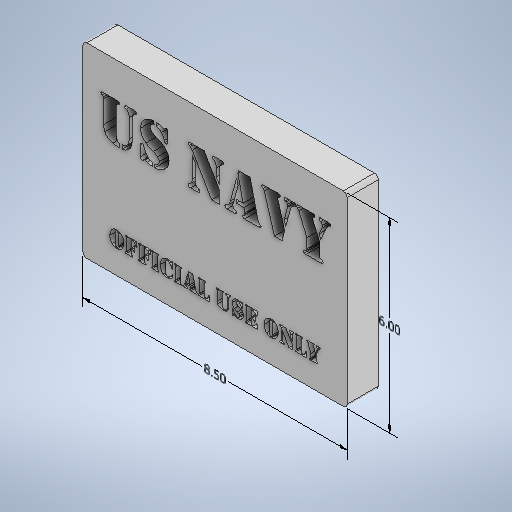
# Autodesk Inventor part: License Plate Stencil
Saved by Autodesk Inventor 2025 (Build 290162000, 162)
## iProperties
Created: 2024-06-17
Part Number: License Plate Stencil
Material: Generic
Document SubType Name: Modeling
Designer: Devon
Density: 1 g/cm^3
Appearance: Default
Author: Devon
Autodesk Inventor part; units mm, degrees
(part 1 of 2)
ref_plane "YZ Plane" through (0, 0, 0) normal (1, 0, 0) x (0, 1, 0)
ref_plane "XZ Plane" through (0, 0, 0) normal (0, 1, 0) x (-1, 0, 0)
ref_plane "XY Plane" through (0, 0, 0) normal (0, 0, 1) x (1, 0, 0)
sketch "Sketch1" plane through (0, 0, 0) normal (0, 0, 1) x (1, 0, 0)
  line L0 (0, 0) -> (304.8, 0)
  line L1 (304.8, 0) -> (304.8, 152.4)
  line L2 (304.8, 152.4) -> (0, 152.4)
  line L3 (0, 152.4) -> (0, 0)
  line L4 (0, 0) -> (44.45, 0)
  line L5 (0, 0) -> (44.45, 0) construction
  line L6 (44.45, 0) -> (44.45, 152.4)
  line L7 (304.8, 0) -> (260.35, 0)
  line L8 (260.35, 0) -> (260.35, 152.4)
  dimension "d0" = 304.8
  dimension "d1" = 152.4
  dimension "d2" = 44.45
  dimension "d3" = 0
  dimension "d4" = 44.45
  constraints: 18 end point, 3 horizontal, 3 perpendicular, 3 point on line, 2 parallel, 1 collinear
  measures "d0" distance of L2.end L1.end
  measures "d1" distance of L1.end L0.end
  measures "d2" distance of L0.start L4.end
  measures "d3" distance between parallel lines of L4 L5
  measures "d4" distance of L0.end L7.end
extrude "Extrusion1" add sketch "Sketch1" along normal blind 25.4 contours L6 L2 L8 L0
fillet "Fillet1" radius 3.175 1 edges at (260.35, 152.4, 12.7)
fillet "Fillet2" radius 3.175 1 edges at (44.45, 152.4, 12.7)
fillet "Fillet3" radius 3.175 1 edges at (260.35, 0, 12.7)
fillet "Fillet4" radius 3.175 1 edges at (44.45, 0, 12.7)
sketch "Sketch2" plane through (0, 0, 25.4) normal (0, 0, 1) x (1, 0, 0)
  line L0 (44.45, 149.225) -> (44.45, 3.175) projected
  line L1 (260.35, 3.175) -> (260.35, 149.225) projected
  line L2 (44.45, 134.9251) -> (260.35, 134.9251) construction
  line L3 (260.35, 134.9251) -> (260.35, 81.3906) construction
  line L4 (260.35, 81.3906) -> (44.45, 81.3906) construction
  line L5 (44.45, 81.3906) -> (44.45, 134.9251) construction
  line L6 (44.45, 46.9482) -> (260.35, 46.9482) construction
  line L7 (260.35, 46.9482) -> (260.35, 4.5325) construction
  line L8 (260.35, 4.5325) -> (44.45, 4.5325) construction
  line L9 (44.45, 4.5325) -> (44.45, 46.9482) construction
  line L10 (61.5459, 101.5708) -> (61.5459, 119.7885)
  spline S0 degree 2 poles (61.5459, 119.7885) (61.5459, 120.6153) (61.2703, 120.9736) knots 0 0 0 1 1 1
  spline S1 degree 2 poles (61.2703, 120.9736) (61.1325, 121.1941) (60.8845, 121.3043) (60.1128, 121.5524) knots 0 0 0 1 2 2 2
  spline S2 degree 2 poles (60.1128, 121.5524) (59.1757, 121.8556) (59.1757, 122.7926) knots 0 0 0 1 1 1
  spline S3 degree 2 poles (59.1757, 122.7926) (59.1757, 123.399) (60.0852, 124.0329) (60.912, 124.0329) knots 0 0 0 1 2 2 2
  line L11 (60.912, 124.0329) -> (61.5184, 124.0329)
  line L12 (61.5184, 124.0329) -> (71.9088, 124.0329)
  line L13 (71.9088, 124.0329) -> (72.5151, 124.0329)
  line L14 (72.5151, 124.0329) -> (73.342, 123.9502)
  spline S4 degree 2 poles (73.342, 123.9502) (73.7278, 123.8124) (74.2515, 123.206) (74.2515, 122.7926) knots 0 0 0 1 2 2 2
  spline S5 degree 2 poles (74.2515, 122.7926) (74.2515, 121.8556) (73.3144, 121.5524) knots 0 0 0 1 1 1
  spline S6 degree 2 poles (73.3144, 121.5524) (72.5427, 121.3043) (72.2946, 121.1941) (72.1568, 120.9736) knots 0 0 0 1 2 2 2
  spline S7 degree 2 poles (72.1568, 120.9736) (71.8812, 120.6153) (71.8812, 119.7885) knots 0 0 0 1 1 1
  line L15 (71.8812, 119.7885) -> (71.8812, 100.2755)
  spline S8 degree 2 poles (71.8812, 100.2755) (71.8812, 98.3187) (72.1017, 96.7477) (72.4049, 96.1138) knots 0 0 0 1 2 2 2
  spline S9 degree 2 poles (72.4049, 96.1138) (72.7081, 95.535) (73.4522, 95.0389) (74.4995, 94.7082) knots 0 0 0 1 2 2 2
  line L16 (74.4995, 94.7082) -> (74.4995, 91.649)
  line L17 (74.4995, 91.649) -> (74.0034, 91.649)
  spline S10 degree 2 poles (74.0034, 91.649) (70.9717, 91.649) (68.9598, 92.2002) knots 0 0 0 1 1 1
  spline S11 degree 2 poles (68.9598, 92.2002) (66.6171, 92.8065) (63.0893, 95.287) (62.3452, 96.8028) knots 0 0 0 1 2 2 2
  spline S12 degree 2 poles (62.3452, 96.8028) (61.5459, 98.4565) (61.5459, 101.5708) knots 0 0 0 1 1 1
  line L18 (76.6492, 91.649) -> (76.6492, 94.7082)
  spline S13 degree 2 poles (76.6492, 94.7082) (78.9643, 95.0114) (80.5353, 96.6099) knots 0 0 0 1 1 1
  spline S14 degree 2 poles (80.5353, 96.6099) (82.2992, 98.4565) (82.2992, 101.874) knots 0 0 0 1 1 1
  line L19 (82.2992, 101.874) -> (82.2992, 117.0324)
  spline S15 degree 2 poles (82.2992, 117.0324) (82.2992, 120.2295) (79.8463, 121.4973) knots 0 0 0 1 1 1
  spline S16 degree 2 poles (79.8463, 121.4973) (79.1297, 121.8556) (78.6887, 122.4068) (78.6887, 122.9029) knots 0 0 0 1 2 2 2
  spline S17 degree 2 poles (78.6887, 122.9029) (78.6887, 123.5092) (79.5707, 124.0329) (80.5904, 124.0329) knots 0 0 0 1 2 2 2
  line L20 (80.5904, 124.0329) -> (86.2679, 124.0329)
  spline S18 degree 2 poles (86.2679, 124.0329) (86.9845, 124.0329) (87.4806, 123.9502) (87.7011, 123.8124) knots 0 0 0 1 2 2 2
  spline S19 degree 2 poles (87.7011, 123.8124) (88.3074, 123.4816) (88.3074, 122.8753) knots 0 0 0 1 1 1
  spline S20 degree 2 poles (88.3074, 122.8753) (88.3074, 122.3517) (87.9492, 121.9934) knots 0 0 0 1 1 1
  spline S21 degree 2 poles (87.9492, 121.9934) (87.8114, 121.8831) (86.9294, 121.387) knots 0 0 0 1 1 1
  spline S22 degree 2 poles (86.9294, 121.387) (85.9097, 120.8083) (84.7521, 118.5207) (84.7521, 117.0324) knots 0 0 0 1 2 2 2
  line L21 (84.7521, 117.0324) -> (84.7521, 101.874)
  spline S23 degree 2 poles (84.7521, 101.874) (84.7521, 97.9604) (83.0433, 95.4523) knots 0 0 0 1 1 1
  spline S24 degree 2 poles (83.0433, 95.4523) (81.7755, 93.5782) (79.4329, 92.4758) knots 0 0 0 1 1 1
  spline S25 degree 2 poles (79.4329, 92.4758) (78.2753, 91.897) (76.6492, 91.649) knots 0 0 0 1 1 1
  line L22 (102.5288, 124.6668) -> (102.5288, 121.9934)
  spline S26 degree 2 poles (102.5288, 121.9934) (101.0956, 121.58) (99.5798, 119.9263) (99.5798, 118.7412) knots 0 0 0 1 2 2 2
  spline S27 degree 2 poles (99.5798, 118.7412) (99.5798, 117.5561) (100.8476, 115.8198) (102.2532, 115.0205) knots 0 0 0 1 2 2 2
  spline S28 degree 2 poles (102.2532, 115.0205) (103.2178, 114.4968) (106.6629, 112.981) knots 0 0 0 1 1 1
  spline S29 degree 2 poles (106.6629, 112.981) (108.7575, 112.0715) (111.0451, 110.6108) (112.0924, 109.5083) knots 0 0 0 1 2 2 2
  spline S30 degree 2 poles (112.0924, 109.5083) (114.8209, 106.642) (114.8209, 102.6457) knots 0 0 0 1 1 1
  spline S31 degree 2 poles (114.8209, 102.6457) (114.8209, 99.6691) (111.8443, 94.6806) (109.2536, 93.2475) knots 0 0 0 1 2 2 2
  spline S32 degree 2 poles (109.2536, 93.2475) (107.848, 92.5033) (104.5132, 91.649) (103.08, 91.649) knots 0 0 0 1 2 2 2
  line L23 (103.08, 91.649) -> (103.08, 94.2948)
  spline S33 degree 2 poles (103.08, 94.2948) (105.092, 94.7909) (106.8834, 96.5272) (106.8834, 98.0155) knots 0 0 0 1 2 2 2
  spline S34 degree 2 poles (106.8834, 98.0155) (106.8834, 99.5865) (105.4778, 100.7716) knots 0 0 0 1 1 1
  spline S35 degree 2 poles (105.4778, 100.7716) (104.5683, 101.5433) (101.95, 102.6733) knots 0 0 0 1 1 1
  spline S36 degree 2 poles (101.95, 102.6733) (99.1113, 103.9411) (96.9891, 105.0159) (95.9969, 105.7325) knots 0 0 0 1 2 2 2
  spline S37 degree 2 poles (95.9969, 105.7325) (91.6423, 108.8469) (91.6423, 114.0283) knots 0 0 0 1 1 1
  spline S38 degree 2 poles (91.6423, 114.0283) (91.6423, 116.6741) (93.8196, 121.1665) (95.7764, 122.5446) knots 0 0 0 1 2 2 2
  spline S39 degree 2 poles (95.7764, 122.5446) (98.5049, 124.4463) (102.5288, 124.6668) knots 0 0 0 1 1 1
  line L24 (101.3161, 94.2948) -> (101.3161, 91.649)
  spline S40 degree 2 poles (101.3161, 91.649) (99.4144, 91.649) (97.0993, 92.7238) knots 0 0 0 1 1 1
  spline S41 degree 2 poles (97.0993, 92.7238) (96.2449, 93.1372) (95.5835, 93.3577) (95.2803, 93.3577) knots 0 0 0 1 2 2 2
  spline S42 degree 2 poles (95.2803, 93.3577) (94.8393, 93.3577) (94.3708, 93.0546) (93.8472, 92.4482) knots 0 0 0 1 2 2 2
  spline S43 degree 2 poles (93.8472, 92.4482) (93.4337, 91.9521) (92.9377, 91.9521) knots 0 0 0 1 1 1
  spline S44 degree 2 poles (92.9377, 91.9521) (91.6423, 91.9521) (91.6423, 93.9641) knots 0 0 0 1 1 1
  line L25 (91.6423, 93.9641) -> (91.6423, 102.4252)
  spline S45 degree 2 poles (91.6423, 102.4252) (91.6423, 103.0591) (92.3864, 103.9686) (92.9377, 103.9962) knots 0 0 0 1 2 2 2
  spline S46 degree 2 poles (92.9377, 103.9962) (93.4613, 104.0237) (94.0401, 103.3898) (94.2606, 102.5906) knots 0 0 0 1 2 2 2
  spline S47 degree 2 poles (94.2606, 102.5906) (94.7842, 100.6062) (96.7962, 97.106) (98.1466, 95.9209) knots 0 0 0 1 2 2 2
  spline S48 degree 2 poles (98.1466, 95.9209) (99.5247, 94.6531) (101.3161, 94.2948) knots 0 0 0 1 1 1
  line L26 (104.3754, 121.9934) -> (104.3754, 124.5565)
  spline S49 degree 2 poles (104.3754, 124.5565) (105.781, 124.4463) (107.8205, 123.8951) (109.6946, 123.0958) knots 0 0 0 1 2 2 2
  spline S50 degree 2 poles (109.6946, 123.0958) (110.1631, 122.9029) (110.4663, 122.9029) knots 0 0 0 1 1 1
  spline S51 degree 2 poles (110.4663, 122.9029) (110.9073, 122.9029) (111.1278, 123.206) knots 0 0 0 1 1 1
  line L27 (111.1278, 123.206) -> (111.6239, 123.8951)
  spline S52 degree 2 poles (111.6239, 123.8951) (112.0097, 124.4187) (112.5334, 124.4187) knots 0 0 0 1 1 1
  spline S53 degree 2 poles (112.5334, 124.4187) (113.1673, 124.4187) (113.746, 123.5092) (113.746, 122.5446) knots 0 0 0 1 2 2 2
  line L28 (113.746, 122.5446) -> (113.746, 114.8551)
  spline S54 degree 2 poles (113.746, 114.8551) (113.746, 114.1661) (112.9743, 113.3117) (112.368, 113.3117) knots 0 0 0 1 2 2 2
  spline S55 degree 2 poles (112.368, 113.3117) (111.8995, 113.3117) (111.5136, 113.6149) knots 0 0 0 1 1 1
  spline S56 degree 2 poles (111.5136, 113.6149) (111.2931, 113.8078) (111.0451, 114.3315) (110.9348, 114.9654) knots 0 0 0 1 2 2 2
  spline S57 degree 2 poles (110.9348, 114.9654) (110.6868, 116.1229) (109.419, 118.5207) (108.5922, 119.4853) knots 0 0 0 1 2 2 2
  spline S58 degree 2 poles (108.5922, 119.4853) (106.911, 121.387) (104.3754, 121.9934) knots 0 0 0 1 1 1
  line L29 (143.5668, 124.0329) -> (155.9416, 102.5355)
  line L30 (155.9416, 102.5355) -> (155.9416, 92.2829)
  line L31 (155.9416, 92.2829) -> (149.6026, 92.2829)
  line L32 (149.6026, 92.2829) -> (133.8103, 119.4853)
  spline S59 degree 2 poles (133.8103, 119.4853) (133.2866, 120.3948) (132.6252, 121.0839) (132.1291, 121.2492) knots 0 0 0 1 2 2 2
  line L33 (132.1291, 121.2492) -> (131.2471, 121.58)
  spline S60 degree 2 poles (131.2471, 121.58) (130.8888, 121.6902) (130.4754, 122.2965) (130.4754, 122.6548) knots 0 0 0 1 2 2 2
  spline S61 degree 2 poles (130.4754, 122.6548) (130.4754, 123.0682) (130.8888, 123.7297) (131.2471, 123.8675) knots 0 0 0 1 2 2 2
  spline S62 degree 2 poles (131.2471, 123.8675) (131.633, 124.0329) (133.3969, 124.0329) knots 0 0 0 1 1 1
  line L34 (133.3969, 124.0329) -> (143.5668, 124.0329)
  line L35 (133.8103, 115.8473) -> (136.2632, 111.7683)
  line L36 (136.2632, 111.7683) -> (136.2632, 99.3109)
  spline S63 degree 2 poles (136.2632, 99.3109) (136.2632, 97.6848) (137.3656, 95.5902) (138.5507, 94.9011) knots 0 0 0 1 2 2 2
  line L37 (138.5507, 94.9011) -> (139.2397, 94.5153)
  spline S64 degree 2 poles (139.2397, 94.5153) (139.8461, 94.157) (139.8461, 93.468) knots 0 0 0 1 1 1
  spline S65 degree 2 poles (139.8461, 93.468) (139.8461, 92.9443) (139.4051, 92.586) knots 0 0 0 1 1 1
  spline S66 degree 2 poles (139.4051, 92.586) (139.0193, 92.2829) (137.8617, 92.2829) knots 0 0 0 1 1 1
  line L38 (137.8617, 92.2829) -> (132.5149, 92.2829)
  spline S67 degree 2 poles (132.5149, 92.2829) (130.3927, 92.2829) (130.3927, 93.4955) knots 0 0 0 1 1 1
  spline S68 degree 2 poles (130.3927, 93.4955) (130.3927, 93.9089) (130.8337, 94.405) (131.5778, 94.8185) knots 0 0 0 1 2 2 2
  spline S69 degree 2 poles (131.5778, 94.8185) (133.8103, 96.0587) (133.8103, 99.3109) knots 0 0 0 1 1 1
  line L39 (133.8103, 99.3109) -> (133.8103, 115.8473)
  line L40 (155.9416, 106.2562) -> (153.4887, 110.4178)
  line L41 (153.4887, 110.4178) -> (153.4887, 116.8671)
  spline S70 degree 2 poles (153.4887, 116.8671) (153.4887, 118.8239) (152.3587, 120.8909) (150.8979, 121.6351) knots 0 0 0 1 2 2 2
  spline S71 degree 2 poles (150.8979, 121.6351) (150.4294, 121.8556) (150.0436, 122.4068) (150.0436, 122.8202) knots 0 0 0 1 2 2 2
  spline S72 degree 2 poles (150.0436, 122.8202) (150.0436, 123.4541) (150.8704, 124.0329) (151.7799, 124.0329) knots 0 0 0 1 2 2 2
  line L42 (151.7799, 124.0329) -> (157.5676, 124.0329)
  spline S73 degree 2 poles (157.5676, 124.0329) (158.7528, 124.0329) (159.1386, 123.647) knots 0 0 0 1 1 1
  spline S74 degree 2 poles (159.1386, 123.647) (159.5245, 123.2887) (159.5245, 122.7651) knots 0 0 0 1 1 1
  spline S75 degree 2 poles (159.5245, 122.7651) (159.5245, 122.2965) (159.0835, 121.8004) (158.2567, 121.387) knots 0 0 0 1 2 2 2
  spline S76 degree 2 poles (158.2567, 121.387) (157.0164, 120.7531) (156.3825, 119.4578) knots 0 0 0 1 1 1
  spline S77 degree 2 poles (156.3825, 119.4578) (155.9416, 118.4931) (155.9416, 116.8671) knots 0 0 0 1 1 1
  line L43 (155.9416, 116.8671) -> (155.9416, 106.2562)
  line L44 (171.7063, 124.0329) -> (181.077, 124.0329)
  line L45 (181.077, 124.0329) -> (187.5262, 96.6926)
  spline S78 degree 2 poles (187.5262, 96.6926) (187.7191, 95.976) (187.9396, 95.4248) knots 0 0 0 1 1 1
  spline S79 degree 2 poles (187.9396, 95.4248) (188.1601, 94.9838) (188.8767, 94.7082) knots 0 0 0 1 1 1
  spline S80 degree 2 poles (188.8767, 94.7082) (189.483, 94.4326) (189.9515, 93.9365) (189.9515, 93.4955) knots 0 0 0 1 2 2 2
  spline S81 degree 2 poles (189.9515, 93.4955) (189.9515, 92.2829) (188.1325, 92.2829) knots 0 0 0 1 1 1
  line L46 (188.1325, 92.2829) -> (176.5294, 92.2829)
  spline S82 degree 2 poles (176.5294, 92.2829) (175.8404, 92.2829) (174.986, 92.9719) (174.986, 93.5231) knots 0 0 0 1 2 2 2
  spline S83 degree 2 poles (174.986, 93.5231) (174.986, 93.9916) (175.3719, 94.4602) (176.0058, 94.7909) knots 0 0 0 1 2 2 2
  spline S84 degree 2 poles (176.0058, 94.7909) (176.4743, 95.0389) (176.8602, 95.5902) (176.8602, 96.0036) knots 0 0 0 1 2 2 2
  spline S85 degree 2 poles (176.8602, 96.0036) (176.8602, 96.417) (176.7775, 96.7201) knots 0 0 0 1 1 1
  line L47 (176.7775, 96.7201) -> (176.0334, 100.0826)
  line L48 (176.0334, 100.0826) -> (169.5566, 100.0826)
  line L49 (169.5566, 100.0826) -> (170.1905, 102.8386)
  line L50 (170.1905, 102.8386) -> (175.3995, 102.8386)
  line L51 (175.3995, 102.8386) -> (171.1, 121.7453)
  line L52 (171.1, 121.7453) -> (171.7063, 124.0329)
  line L53 (170.0802, 118.1073) -> (171.2653, 113.3117)
  line L54 (171.2653, 113.3117) -> (167.1588, 98.2911)
  spline S86 degree 2 poles (167.1588, 98.2911) (166.9659, 97.6296) (166.9659, 97.0784) knots 0 0 0 1 1 1
  spline S87 degree 2 poles (166.9659, 97.0784) (166.9659, 95.6177) (168.3439, 94.9838) knots 0 0 0 1 1 1
  line L55 (168.3439, 94.9838) -> (169.1432, 94.598)
  spline S88 degree 2 poles (169.1432, 94.598) (169.9149, 94.2672) (169.9149, 93.4404) knots 0 0 0 1 1 1
  spline S89 degree 2 poles (169.9149, 93.4404) (169.9149, 92.2829) (168.2337, 92.2829) knots 0 0 0 1 1 1
  line L56 (168.2337, 92.2829) -> (162.3357, 92.2829)
  spline S90 degree 2 poles (162.3357, 92.2829) (161.4537, 92.2829) (160.4615, 92.9994) (160.4615, 93.6333) knots 0 0 0 1 2 2 2
  spline S91 degree 2 poles (160.4615, 93.6333) (160.4615, 94.2948) (161.4813, 94.7358) knots 0 0 0 1 1 1
  spline S92 degree 2 poles (161.4813, 94.7358) (162.4459, 95.1767) (163.3554, 95.8382) (163.7688, 96.417) knots 0 0 0 1 2 2 2
  spline S93 degree 2 poles (163.7688, 96.417) (164.4027, 97.3816) (164.8437, 98.9526) knots 0 0 0 1 1 1
  line L57 (164.8437, 98.9526) -> (170.0802, 118.1073)
  line L58 (209.2441, 100.4133) -> (207.0392, 92.2829)
  line L59 (207.0392, 92.2829) -> (200.9207, 92.2829)
  line L60 (200.9207, 92.2829) -> (192.6525, 120.0917)
  spline S94 degree 2 poles (192.6525, 120.0917) (192.4596, 120.698) (192.1564, 121.139) (191.7981, 121.3043) knots 0 0 0 1 2 2 2
  spline S95 degree 2 poles (191.7981, 121.3043) (191.054, 121.6075) (190.5854, 122.1312) (190.5854, 122.6273) knots 0 0 0 1 2 2 2
  spline S96 degree 2 poles (190.5854, 122.6273) (190.5854, 123.3438) (191.2193, 123.7297) knots 0 0 0 1 1 1
  spline S97 degree 2 poles (191.2193, 123.7297) (191.6879, 124.0329) (192.8179, 124.0329) knots 0 0 0 1 1 1
  line L61 (192.8179, 124.0329) -> (203.1531, 124.0329)
  spline S98 degree 2 poles (203.1531, 124.0329) (204.1453, 124.0329) (204.8619, 123.9502) (205.11, 123.8124) knots 0 0 0 1 2 2 2
  spline S99 degree 2 poles (205.11, 123.8124) (205.3304, 123.647) (205.6612, 123.0407) (205.6612, 122.7651) knots 0 0 0 1 2 2 2
  spline S100 degree 2 poles (205.6612, 122.7651) (205.6612, 121.8831) (204.8344, 121.5248) knots 0 0 0 1 1 1
  spline S101 degree 2 poles (204.8344, 121.5248) (204.228, 121.2217) (203.787, 120.5878) (203.787, 120.009) knots 0 0 0 1 2 2 2
  spline S102 degree 2 poles (203.787, 120.009) (203.787, 119.6231) (203.8697, 119.3475) knots 0 0 0 1 1 1
  line L62 (203.8697, 119.3475) -> (209.2441, 100.4133)
  line L63 (210.126, 103.7481) -> (208.9133, 108.1027)
  line L64 (208.9133, 108.1027) -> (211.5867, 117.9144)
  spline S103 degree 2 poles (211.5867, 117.9144) (211.8348, 118.8514) (211.8623, 119.0444) knots 0 0 0 1 1 1
  spline S104 degree 2 poles (211.8623, 119.0444) (211.9175, 119.568) (211.6419, 120.2019) knots 0 0 0 1 1 1
  spline S105 degree 2 poles (211.6419, 120.2019) (211.256, 121.0012) (210.4567, 121.2768) knots 0 0 0 1 1 1
  line L65 (210.4567, 121.2768) -> (209.685, 121.5524)
  spline S106 degree 2 poles (209.685, 121.5524) (208.7755, 121.8556) (208.7755, 122.7375) knots 0 0 0 1 1 1
  spline S107 degree 2 poles (208.7755, 122.7375) (208.7755, 123.3714) (209.7953, 124.0329) (210.7048, 124.0329) knots 0 0 0 1 2 2 2
  line L66 (210.7048, 124.0329) -> (216.4099, 124.0329)
  spline S108 degree 2 poles (216.4099, 124.0329) (217.4847, 124.0329) (217.8155, 123.8124) knots 0 0 0 1 1 1
  spline S109 degree 2 poles (217.8155, 123.8124) (218.3667, 123.4816) (218.3667, 122.8202) knots 0 0 0 1 1 1
  spline S110 degree 2 poles (218.3667, 122.8202) (218.3667, 122.3792) (218.0084, 121.8556) (217.5399, 121.6626) knots 0 0 0 1 2 2 2
  line L67 (217.5399, 121.6626) -> (216.3548, 121.1114)
  spline S111 degree 2 poles (216.3548, 121.1114) (215.6106, 120.7531) (214.2601, 118.6861) (213.8743, 117.3632) knots 0 0 0 1 2 2 2
  line L68 (213.8743, 117.3632) -> (210.126, 103.7481)
  line L69 (237.797, 106.8349) -> (237.797, 96.6926)
  spline S112 degree 2 poles (237.797, 96.6926) (237.797, 95.7831) (238.1553, 95.3972) knots 0 0 0 1 1 1
  spline S113 degree 2 poles (238.1553, 95.3972) (238.3207, 95.1767) (238.6514, 95.0389) (239.5609, 94.8185) knots 0 0 0 1 2 2 2
  spline S114 degree 2 poles (239.5609, 94.8185) (240.6909, 94.5704) (240.6909, 93.5507) knots 0 0 0 1 1 1
  spline S115 degree 2 poles (240.6909, 93.5507) (240.6909, 92.8616) (240.057, 92.5033) knots 0 0 0 1 1 1
  spline S116 degree 2 poles (240.057, 92.5033) (239.6987, 92.2829) (238.6238, 92.2829) knots 0 0 0 1 1 1
  line L70 (238.6238, 92.2829) -> (237.8246, 92.2829)
  line L71 (237.8246, 92.2829) -> (227.4342, 92.2829)
  line L72 (227.4342, 92.2829) -> (226.6625, 92.2829)
  spline S117 degree 2 poles (226.6625, 92.2829) (225.6152, 92.2829) (225.2018, 92.5585) knots 0 0 0 1 1 1
  spline S118 degree 2 poles (225.2018, 92.5585) (224.5954, 92.9443) (224.5954, 93.5507) knots 0 0 0 1 1 1
  spline S119 degree 2 poles (224.5954, 93.5507) (224.5954, 94.5704) (225.7254, 94.8185) knots 0 0 0 1 1 1
  spline S120 degree 2 poles (225.7254, 94.8185) (226.6349, 95.0389) (226.9381, 95.1767) (227.1035, 95.3972) knots 0 0 0 1 2 2 2
  spline S121 degree 2 poles (227.1035, 95.3972) (227.4617, 95.7831) (227.4617, 96.6926) knots 0 0 0 1 1 1
  line L73 (227.4617, 96.6926) -> (227.4617, 104.5474)
  line L74 (227.4617, 104.5474) -> (220.8747, 120.257)
  spline S122 degree 2 poles (220.8747, 120.257) (220.5164, 121.139) (219.8274, 121.5524) knots 0 0 0 1 1 1
  spline S123 degree 2 poles (219.8274, 121.5524) (219.2211, 121.9382) (218.8628, 122.4068) (218.8628, 122.8202) knots 0 0 0 1 2 2 2
  spline S124 degree 2 poles (218.8628, 122.8202) (218.8628, 124.0329) (220.6267, 124.0329) knots 0 0 0 1 1 1
  line L75 (220.6267, 124.0329) -> (232.0368, 124.0329)
  spline S125 degree 2 poles (232.0368, 124.0329) (232.9188, 124.0329) (233.2771, 123.8124) knots 0 0 0 1 1 1
  spline S126 degree 2 poles (233.2771, 123.8124) (233.8558, 123.4541) (233.8558, 122.8477) knots 0 0 0 1 1 1
  spline S127 degree 2 poles (233.8558, 122.8477) (233.8558, 122.1036) (233.1944, 121.6902) knots 0 0 0 1 1 1
  line L76 (233.1944, 121.6902) -> (232.5054, 121.2768)
  spline S128 degree 2 poles (232.5054, 121.2768) (232.1195, 121.0012) (232.1195, 120.5051) knots 0 0 0 1 1 1
  spline S129 degree 2 poles (232.1195, 120.5051) (232.1195, 119.9263) (232.3676, 119.3475) knots 0 0 0 1 1 1
  line L77 (232.3676, 119.3475) -> (237.797, 106.8349)
  line L78 (238.7065, 109.0398) -> (237.3836, 112.0991)
  line L79 (237.3836, 112.0991) -> (239.8365, 117.5561)
  spline S130 degree 2 poles (239.8365, 117.5561) (240.1397, 118.2727) (240.1397, 119.4578) knots 0 0 0 1 1 1
  spline S131 degree 2 poles (240.1397, 119.4578) (240.1397, 120.8083) (238.6514, 121.4146) knots 0 0 0 1 1 1
  spline S132 degree 2 poles (238.6514, 121.4146) (237.8521, 121.7178) (237.3561, 122.2139) (237.3561, 122.7375) knots 0 0 0 1 2 2 2
  spline S133 degree 2 poles (237.3561, 122.7375) (237.3561, 123.3714) (237.7695, 123.6746) knots 0 0 0 1 1 1
  spline S134 degree 2 poles (237.7695, 123.6746) (238.0451, 123.8951) (238.7341, 124.0329) (239.616, 124.0329) knots 0 0 0 1 2 2 2
  line L80 (239.616, 124.0329) -> (245.3487, 124.0329)
  spline S135 degree 2 poles (245.3487, 124.0329) (246.9748, 124.0329) (246.9748, 122.7375) knots 0 0 0 1 1 1
  spline S136 degree 2 poles (246.9748, 122.7375) (246.9748, 122.269) (246.5338, 121.7453) (245.8999, 121.4697) knots 0 0 0 1 2 2 2
  spline S137 degree 2 poles (245.8999, 121.4697) (244.7699, 120.9736) (244.2738, 120.45) knots 0 0 0 1 1 1
  spline S138 degree 2 poles (244.2738, 120.45) (243.5848, 119.7058) (243.1163, 118.7412) knots 0 0 0 1 1 1
  line L81 (243.1163, 118.7412) -> (242.5926, 117.5561)
  line L82 (242.5926, 117.5561) -> (238.7065, 109.0398)
  line L83 (72.551, 31.3407) -> (72.551, 32.3439)
  spline S139 degree 2 poles (72.551, 32.3439) (73.5542, 32.2998) (75.2188, 31.5722) (75.9354, 30.8667) knots 0 0 0 1 2 2 2
  spline S140 degree 2 poles (75.9354, 30.8667) (77.8316, 29.0146) (77.8316, 25.7293) knots 0 0 0 1 1 1
  spline S141 degree 2 poles (77.8316, 25.7293) (77.8316, 22.4992) (76.0236, 20.6912) knots 0 0 0 1 1 1
  spline S142 degree 2 poles (76.0236, 20.6912) (74.6235, 19.3022) (72.551, 19.1368) knots 0 0 0 1 1 1
  line L84 (72.551, 19.1368) -> (72.551, 20.162)
  spline S143 degree 2 poles (72.551, 20.162) (72.7935, 20.2172) (73.0581, 20.3936) (73.1683, 20.5589) knots 0 0 0 1 2 2 2
  spline S144 degree 2 poles (73.1683, 20.5589) (73.4219, 20.9448) (73.4219, 21.7165) knots 0 0 0 1 1 1
  line L85 (73.4219, 21.7165) -> (73.4219, 30.0288)
  spline S145 degree 2 poles (73.4219, 30.0288) (73.4219, 30.5249) (73.2565, 30.8115) knots 0 0 0 1 1 1
  spline S146 degree 2 poles (73.2565, 30.8115) (73.1463, 31.01) (72.8376, 31.2305) (72.551, 31.3407) knots 0 0 0 1 2 2 2
  spline S147 degree 2 poles (71.7903, 31.3407) (71.3162, 31.1643) (70.9304, 30.591) (70.9304, 30.0288) knots 0 0 0 1 2 2 2
  line L86 (70.9304, 30.0288) -> (70.9304, 21.7165)
  spline S148 degree 2 poles (70.9304, 21.7165) (70.9304, 20.9007) (71.1509, 20.5589) knots 0 0 0 1 1 1
  spline S149 degree 2 poles (71.1509, 20.5589) (71.3273, 20.2833) (71.7903, 20.162) knots 0 0 0 1 1 1
  line L87 (71.7903, 20.162) -> (71.7903, 19.1368)
  spline S150 degree 2 poles (71.7903, 19.1368) (69.7287, 19.3022) (68.3286, 20.6912) knots 0 0 0 1 1 1
  spline S151 degree 2 poles (68.3286, 20.6912) (66.5207, 22.4992) (66.5207, 25.7293) knots 0 0 0 1 1 1
  spline S152 degree 2 poles (66.5207, 25.7293) (66.5207, 27.3499) (67.4798, 29.9627) (68.4168, 30.8667) knots 0 0 0 1 2 2 2
  spline S153 degree 2 poles (68.4168, 30.8667) (69.1334, 31.5722) (70.7871, 32.2998) (71.7903, 32.3439) knots 0 0 0 1 2 2 2
  line L88 (71.7903, 32.3439) -> (71.7903, 31.3407)
  line L89 (84.0603, 32.0903) -> (84.0603, 21.1542)
  spline S154 degree 2 poles (84.0603, 21.1542) (84.0603, 20.7904) (84.2036, 20.6361) knots 0 0 0 1 1 1
  spline S155 degree 2 poles (84.2036, 20.6361) (84.2698, 20.5479) (84.4021, 20.4928) (84.7659, 20.4046) knots 0 0 0 1 2 2 2
  spline S156 degree 2 poles (84.7659, 20.4046) (85.2179, 20.3054) (85.2179, 19.8975) knots 0 0 0 1 1 1
  spline S157 degree 2 poles (85.2179, 19.8975) (85.2179, 19.6549) (84.9753, 19.5006) knots 0 0 0 1 1 1
  spline S158 degree 2 poles (84.9753, 19.5006) (84.799, 19.3903) (84.3911, 19.3903) knots 0 0 0 1 1 1
  line L90 (84.3911, 19.3903) -> (84.0714, 19.3903)
  line L91 (84.0714, 19.3903) -> (79.9152, 19.3903)
  line L92 (79.9152, 19.3903) -> (79.6727, 19.3903)
  spline S159 degree 2 poles (79.6727, 19.3903) (79.3419, 19.3903) (78.9781, 19.6439) (78.9781, 19.8754) knots 0 0 0 1 2 2 2
  spline S160 degree 2 poles (78.9781, 19.8754) (78.9781, 20.2502) (79.353, 20.3715) knots 0 0 0 1 1 1
  spline S161 degree 2 poles (79.353, 20.3715) (79.6616, 20.4818) (79.7608, 20.5259) (79.816, 20.614) knots 0 0 0 1 2 2 2
  spline S162 degree 2 poles (79.816, 20.614) (79.9262, 20.7574) (79.9262, 21.0881) knots 0 0 0 1 1 1
  line L93 (79.9262, 21.0881) -> (79.9262, 30.3926)
  spline S163 degree 2 poles (79.9262, 30.3926) (79.9262, 30.7233) (79.816, 30.8667) knots 0 0 0 1 1 1
  spline S164 degree 2 poles (79.816, 30.8667) (79.7608, 30.9548) (79.6616, 30.9989) (79.353, 31.0982) knots 0 0 0 1 2 2 2
  spline S165 degree 2 poles (79.353, 31.0982) (78.9781, 31.2194) (78.9781, 31.6053) knots 0 0 0 1 1 1
  spline S166 degree 2 poles (78.9781, 31.6053) (78.9781, 31.8368) (79.3419, 32.0903) (79.6727, 32.0903) knots 0 0 0 1 2 2 2
  line L94 (79.6727, 32.0903) -> (79.9152, 32.0903)
  line L95 (79.9152, 32.0903) -> (84.0603, 32.0903)
  line L96 (84.8761, 32.0903) -> (88.6244, 32.0903)
  line L97 (88.6244, 32.0903) -> (88.6244, 28.8382)
  spline S167 degree 2 poles (88.6244, 28.8382) (88.6244, 28.5295) (88.4039, 28.2539) (88.1503, 28.2539) knots 0 0 0 1 2 2 2
  spline S168 degree 2 poles (88.1503, 28.2539) (87.9629, 28.2539) (87.7535, 28.4523) (87.6763, 28.6838) knots 0 0 0 1 2 2 2
  spline S169 degree 2 poles (87.6763, 28.6838) (87.533, 29.1358) (87.092, 29.8965) (86.8054, 30.1611) knots 0 0 0 1 2 2 2
  spline S170 degree 2 poles (86.8054, 30.1611) (86.4306, 30.5359) (85.5155, 30.9218) (84.8761, 30.9989) knots 0 0 0 1 2 2 2
  line L98 (84.8761, 30.9989) -> (84.8761, 32.0903)
  line L99 (84.832, 25.3104) -> (84.832, 26.3908)
  spline S171 degree 2 poles (84.832, 26.3908) (85.3832, 26.6554) (85.8904, 27.2617) (86.0116, 27.7798) knots 0 0 0 1 2 2 2
  spline S172 degree 2 poles (86.0116, 27.7798) (86.0888, 28.1326) (86.3313, 28.4082) (86.5518, 28.4082) knots 0 0 0 1 2 2 2
  spline S173 degree 2 poles (86.5518, 28.4082) (86.8495, 28.4082) (86.9597, 28.1767) knots 0 0 0 1 1 1
  spline S174 degree 2 poles (86.9597, 28.1767) (87.0259, 28.0555) (87.0259, 27.6255) knots 0 0 0 1 1 1
  line L100 (87.0259, 27.6255) -> (87.0259, 24.0757)
  spline S175 degree 2 poles (87.0259, 24.0757) (87.0259, 23.6347) (86.8274, 23.304) (86.5739, 23.304) knots 0 0 0 1 2 2 2
  spline S176 degree 2 poles (86.5739, 23.304) (86.3534, 23.304) (86.1108, 23.5686) (86.0447, 23.8772) knots 0 0 0 1 2 2 2
  spline S177 degree 2 poles (86.0447, 23.8772) (85.8683, 24.5167) (85.2951, 25.2002) (84.832, 25.3104) knots 0 0 0 1 2 2 2
  line L101 (94.8531, 32.0903) -> (94.8531, 21.1542)
  spline S178 degree 2 poles (94.8531, 21.1542) (94.8531, 20.7904) (94.9964, 20.6361) knots 0 0 0 1 1 1
  spline S179 degree 2 poles (94.9964, 20.6361) (95.0626, 20.5479) (95.1949, 20.4928) (95.5587, 20.4046) knots 0 0 0 1 2 2 2
  spline S180 degree 2 poles (95.5587, 20.4046) (96.0107, 20.3054) (96.0107, 19.8975) knots 0 0 0 1 1 1
  spline S181 degree 2 poles (96.0107, 19.8975) (96.0107, 19.6549) (95.7681, 19.5006) knots 0 0 0 1 1 1
  spline S182 degree 2 poles (95.7681, 19.5006) (95.5918, 19.3903) (95.1839, 19.3903) knots 0 0 0 1 1 1
  line L102 (95.1839, 19.3903) -> (94.8641, 19.3903)
  line L103 (94.8641, 19.3903) -> (90.708, 19.3903)
  line L104 (90.708, 19.3903) -> (90.4654, 19.3903)
  spline S183 degree 2 poles (90.4654, 19.3903) (90.1347, 19.3903) (89.7709, 19.6439) (89.7709, 19.8754) knots 0 0 0 1 2 2 2
  spline S184 degree 2 poles (89.7709, 19.8754) (89.7709, 20.2502) (90.1457, 20.3715) knots 0 0 0 1 1 1
  spline S185 degree 2 poles (90.1457, 20.3715) (90.4544, 20.4818) (90.5536, 20.5259) (90.6088, 20.614) knots 0 0 0 1 2 2 2
  spline S186 degree 2 poles (90.6088, 20.614) (90.719, 20.7574) (90.719, 21.0881) knots 0 0 0 1 1 1
  line L105 (90.719, 21.0881) -> (90.719, 30.3926)
  spline S187 degree 2 poles (90.719, 30.3926) (90.719, 30.7233) (90.6088, 30.8667) knots 0 0 0 1 1 1
  spline S188 degree 2 poles (90.6088, 30.8667) (90.5536, 30.9548) (90.4544, 30.9989) (90.1457, 31.0982) knots 0 0 0 1 2 2 2
  spline S189 degree 2 poles (90.1457, 31.0982) (89.7709, 31.2194) (89.7709, 31.6053) knots 0 0 0 1 1 1
  spline S190 degree 2 poles (89.7709, 31.6053) (89.7709, 31.8368) (90.1347, 32.0903) (90.4654, 32.0903) knots 0 0 0 1 2 2 2
  line L106 (90.4654, 32.0903) -> (90.708, 32.0903)
  line L107 (90.708, 32.0903) -> (94.8531, 32.0903)
  line L108 (95.6689, 32.0903) -> (99.4172, 32.0903)
  line L109 (99.4172, 32.0903) -> (99.4172, 28.8382)
  spline S191 degree 2 poles (99.4172, 28.8382) (99.4172, 28.5295) (99.1967, 28.2539) (98.9431, 28.2539) knots 0 0 0 1 2 2 2
  spline S192 degree 2 poles (98.9431, 28.2539) (98.7557, 28.2539) (98.5463, 28.4523) (98.4691, 28.6838) knots 0 0 0 1 2 2 2
  spline S193 degree 2 poles (98.4691, 28.6838) (98.3258, 29.1358) (97.8848, 29.8965) (97.5982, 30.1611) knots 0 0 0 1 2 2 2
  spline S194 degree 2 poles (97.5982, 30.1611) (97.2233, 30.5359) (96.3083, 30.9218) (95.6689, 30.9989) knots 0 0 0 1 2 2 2
  line L110 (95.6689, 30.9989) -> (95.6689, 32.0903)
  line L111 (95.6248, 25.3104) -> (95.6248, 26.3908)
  spline S195 degree 2 poles (95.6248, 26.3908) (96.176, 26.6554) (96.6832, 27.2617) (96.8044, 27.7798) knots 0 0 0 1 2 2 2
  spline S196 degree 2 poles (96.8044, 27.7798) (96.8816, 28.1326) (97.1241, 28.4082) (97.3446, 28.4082) knots 0 0 0 1 2 2 2
  spline S197 degree 2 poles (97.3446, 28.4082) (97.6423, 28.4082) (97.7525, 28.1767) knots 0 0 0 1 1 1
  spline S198 degree 2 poles (97.7525, 28.1767) (97.8187, 28.0555) (97.8187, 27.6255) knots 0 0 0 1 1 1
  line L112 (97.8187, 27.6255) -> (97.8187, 24.0757)
  spline S199 degree 2 poles (97.8187, 24.0757) (97.8187, 23.6347) (97.6202, 23.304) (97.3667, 23.304) knots 0 0 0 1 2 2 2
  spline S200 degree 2 poles (97.3667, 23.304) (97.1462, 23.304) (96.9036, 23.5686) (96.8375, 23.8772) knots 0 0 0 1 2 2 2
  spline S201 degree 2 poles (96.8375, 23.8772) (96.6611, 24.5167) (96.0878, 25.2002) (95.6248, 25.3104) knots 0 0 0 1 2 2 2
  line L113 (105.6569, 19.3903) -> (101.5008, 19.3903)
  line L114 (101.5008, 19.3903) -> (101.2582, 19.3903)
  spline S202 degree 2 poles (101.2582, 19.3903) (100.9275, 19.3903) (100.5637, 19.6439) (100.5637, 19.8754) knots 0 0 0 1 2 2 2
  spline S203 degree 2 poles (100.5637, 19.8754) (100.5637, 20.2502) (100.9385, 20.3715) knots 0 0 0 1 1 1
  spline S204 degree 2 poles (100.9385, 20.3715) (101.2472, 20.4818) (101.3464, 20.5259) (101.4016, 20.614) knots 0 0 0 1 2 2 2
  spline S205 degree 2 poles (101.4016, 20.614) (101.5118, 20.7574) (101.5118, 21.0881) knots 0 0 0 1 1 1
  line L115 (101.5118, 21.0881) -> (101.5118, 30.3926)
  spline S206 degree 2 poles (101.5118, 30.3926) (101.5118, 30.7233) (101.4016, 30.8667) knots 0 0 0 1 1 1
  spline S207 degree 2 poles (101.4016, 30.8667) (101.3464, 30.9548) (101.2472, 30.9989) (100.9385, 31.0982) knots 0 0 0 1 2 2 2
  spline S208 degree 2 poles (100.9385, 31.0982) (100.5637, 31.2194) (100.5637, 31.6053) knots 0 0 0 1 1 1
  spline S209 degree 2 poles (100.5637, 31.6053) (100.5637, 31.8368) (100.9275, 32.0903) (101.2582, 32.0903) knots 0 0 0 1 2 2 2
  line L116 (101.2582, 32.0903) -> (101.5008, 32.0903)
  line L117 (101.5008, 32.0903) -> (105.6569, 32.0903)
  line L118 (105.6569, 32.0903) -> (105.8995, 32.0903)
  spline S210 degree 2 poles (105.8995, 32.0903) (106.2302, 32.0903) (106.594, 31.8368) (106.594, 31.6053) knots 0 0 0 1 2 2 2
  spline S211 degree 2 poles (106.594, 31.6053) (106.594, 31.2194) (106.2192, 31.0982) knots 0 0 0 1 1 1
  spline S212 degree 2 poles (106.2192, 31.0982) (105.9105, 30.9989) (105.8113, 30.9548) (105.7562, 30.8667) knots 0 0 0 1 2 2 2
  spline S213 degree 2 poles (105.7562, 30.8667) (105.6459, 30.7233) (105.6459, 30.3926) knots 0 0 0 1 1 1
  line L119 (105.6459, 30.3926) -> (105.6459, 21.0881)
  spline S214 degree 2 poles (105.6459, 21.0881) (105.6459, 20.7574) (105.7562, 20.614) knots 0 0 0 1 1 1
  spline S215 degree 2 poles (105.7562, 20.614) (105.8113, 20.5259) (105.9105, 20.4818) (106.2192, 20.3715) knots 0 0 0 1 2 2 2
  spline S216 degree 2 poles (106.2192, 20.3715) (106.594, 20.2502) (106.594, 19.8754) knots 0 0 0 1 1 1
  spline S217 degree 2 poles (106.594, 19.8754) (106.594, 19.6439) (106.2302, 19.3903) (105.8995, 19.3903) knots 0 0 0 1 2 2 2
  line L120 (105.8995, 19.3903) -> (105.6569, 19.3903)
  line L121 (113.2306, 32.3439) -> (113.2306, 31.2194)
  spline S218 degree 2 poles (113.2306, 31.2194) (112.6904, 31.1312) (112.1503, 30.3265) (112.1503, 29.5878) knots 0 0 0 1 2 2 2
  line L122 (112.1503, 29.5878) -> (112.1503, 21.9039)
  line L123 (112.1503, 21.9039) -> (112.1503, 21.496)
  spline S219 degree 2 poles (112.1503, 21.496) (112.1503, 21.2865) (112.3266, 20.8125) (112.4589, 20.6471) knots 0 0 0 1 2 2 2
  spline S220 degree 2 poles (112.4589, 20.6471) (112.6133, 20.4597) (112.944, 20.3054) (113.2306, 20.2723) knots 0 0 0 1 2 2 2
  line L124 (113.2306, 20.2723) -> (113.2306, 19.1368)
  spline S221 degree 2 poles (113.2306, 19.1368) (111.4337, 19.1368) (110.0997, 20.0739) knots 0 0 0 1 1 1
  spline S222 degree 2 poles (110.0997, 20.0739) (108.9312, 20.9007) (107.7405, 23.7009) (107.7405, 25.6191) knots 0 0 0 1 2 2 2
  spline S223 degree 2 poles (107.7405, 25.6191) (107.7405, 27.0302) (108.5122, 29.4555) (109.2509, 30.3485) knots 0 0 0 1 2 2 2
  spline S224 degree 2 poles (109.2509, 30.3485) (109.9895, 31.2415) (112.0621, 32.3439) (113.0212, 32.3439) knots 0 0 0 1 2 2 2
  line L125 (113.0212, 32.3439) -> (113.2306, 32.3439)
  line L126 (113.9693, 31.2084) -> (113.9693, 32.3329)
  spline S225 degree 2 poles (113.9693, 32.3329) (114.4213, 32.2557) (114.9945, 32.0903) (115.7332, 31.8147) knots 0 0 0 1 2 2 2
  spline S226 degree 2 poles (115.7332, 31.8147) (116.2072, 31.6494) (116.3726, 31.6494) knots 0 0 0 1 1 1
  spline S227 degree 2 poles (116.3726, 31.6494) (116.6372, 31.6494) (116.7805, 31.8919) knots 0 0 0 1 1 1
  line L127 (116.7805, 31.8919) -> (116.9017, 32.1234)
  spline S228 degree 2 poles (116.9017, 32.1234) (117.012, 32.3439) (117.3207, 32.3439) knots 0 0 0 1 1 1
  spline S229 degree 2 poles (117.3207, 32.3439) (117.5742, 32.3439) (117.8388, 32.0463) (117.8388, 31.7596) knots 0 0 0 1 2 2 2
  line L128 (117.8388, 31.7596) -> (117.8388, 27.8791)
  spline S230 degree 2 poles (117.8388, 27.8791) (117.8388, 27.5042) (117.6734, 27.3389) knots 0 0 0 1 1 1
  spline S231 degree 2 poles (117.6734, 27.3389) (117.5081, 27.1735) (117.2876, 27.1735) knots 0 0 0 1 1 1
  spline S232 degree 2 poles (117.2876, 27.1735) (117.0671, 27.1735) (116.8025, 27.4601) (116.7143, 27.7909) knots 0 0 0 1 2 2 2
  spline S233 degree 2 poles (116.7143, 27.7909) (116.5159, 28.5185) (116.3285, 28.9374) knots 0 0 0 1 1 1
  spline S234 degree 2 poles (116.3285, 28.9374) (115.9316, 29.8304) (115.4245, 30.3816) knots 0 0 0 1 1 1
  spline S235 degree 2 poles (115.4245, 30.3816) (115.0717, 30.7454) (114.3882, 31.1533) (113.9693, 31.2084) knots 0 0 0 1 2 2 2
  line L129 (113.9913, 19.1368) -> (113.9913, 20.2723)
  spline S236 degree 2 poles (113.9913, 20.2723) (114.7189, 20.3274) (115.5127, 20.8235) knots 0 0 0 1 1 1
  spline S237 degree 2 poles (115.5127, 20.8235) (115.9426, 21.0881) (116.6151, 21.9921) (116.7805, 22.5323) knots 0 0 0 1 2 2 2
  spline S238 degree 2 poles (116.7805, 22.5323) (116.8687, 22.8299) (117.1222, 23.0835) (117.3317, 23.0835) knots 0 0 0 1 2 2 2
  spline S239 degree 2 poles (117.3317, 23.0835) (117.5522, 23.0835) (117.8498, 22.7528) (117.8498, 22.4992) knots 0 0 0 1 2 2 2
  spline S240 degree 2 poles (117.8498, 22.4992) (117.8498, 22.0803) (117.2104, 20.8897) (116.7033, 20.3825) knots 0 0 0 1 2 2 2
  spline S241 degree 2 poles (116.7033, 20.3825) (116.097, 19.7762) (114.7961, 19.1809) (113.9913, 19.1368) knots 0 0 0 1 2 2 2
  line L130 (124.3431, 19.3903) -> (120.187, 19.3903)
  line L131 (120.187, 19.3903) -> (119.9444, 19.3903)
  spline S242 degree 2 poles (119.9444, 19.3903) (119.6137, 19.3903) (119.2499, 19.6439) (119.2499, 19.8754) knots 0 0 0 1 2 2 2
  spline S243 degree 2 poles (119.2499, 19.8754) (119.2499, 20.2502) (119.6247, 20.3715) knots 0 0 0 1 1 1
  spline S244 degree 2 poles (119.6247, 20.3715) (119.9334, 20.4818) (120.0326, 20.5259) (120.0878, 20.614) knots 0 0 0 1 2 2 2
  spline S245 degree 2 poles (120.0878, 20.614) (120.198, 20.7574) (120.198, 21.0881) knots 0 0 0 1 1 1
  line L132 (120.198, 21.0881) -> (120.198, 30.3926)
  spline S246 degree 2 poles (120.198, 30.3926) (120.198, 30.7233) (120.0878, 30.8667) knots 0 0 0 1 1 1
  spline S247 degree 2 poles (120.0878, 30.8667) (120.0326, 30.9548) (119.9334, 30.9989) (119.6247, 31.0982) knots 0 0 0 1 2 2 2
  spline S248 degree 2 poles (119.6247, 31.0982) (119.2499, 31.2194) (119.2499, 31.6053) knots 0 0 0 1 1 1
  spline S249 degree 2 poles (119.2499, 31.6053) (119.2499, 31.8368) (119.6137, 32.0903) (119.9444, 32.0903) knots 0 0 0 1 2 2 2
  line L133 (119.9444, 32.0903) -> (120.187, 32.0903)
  line L134 (120.187, 32.0903) -> (124.3431, 32.0903)
  line L135 (124.3431, 32.0903) -> (124.5857, 32.0903)
  spline S250 degree 2 poles (124.5857, 32.0903) (124.9164, 32.0903) (125.2802, 31.8368) (125.2802, 31.6053) knots 0 0 0 1 2 2 2
  spline S251 degree 2 poles (125.2802, 31.6053) (125.2802, 31.2194) (124.9054, 31.0982) knots 0 0 0 1 1 1
  spline S252 degree 2 poles (124.9054, 31.0982) (124.5967, 30.9989) (124.4975, 30.9548) (124.4424, 30.8667) knots 0 0 0 1 2 2 2
  spline S253 degree 2 poles (124.4424, 30.8667) (124.3321, 30.7233) (124.3321, 30.3926) knots 0 0 0 1 1 1
  line L136 (124.3321, 30.3926) -> (124.3321, 21.0881)
  spline S254 degree 2 poles (124.3321, 21.0881) (124.3321, 20.7574) (124.4424, 20.614) knots 0 0 0 1 1 1
  spline S255 degree 2 poles (124.4424, 20.614) (124.4975, 20.5259) (124.5967, 20.4818) (124.9054, 20.3715) knots 0 0 0 1 2 2 2
  spline S256 degree 2 poles (124.9054, 20.3715) (125.2802, 20.2502) (125.2802, 19.8754) knots 0 0 0 1 1 1
  spline S257 degree 2 poles (125.2802, 19.8754) (125.2802, 19.6439) (124.9164, 19.3903) (124.5857, 19.3903) knots 0 0 0 1 2 2 2
  line L137 (124.5857, 19.3903) -> (124.3431, 19.3903)
  line L138 (130.5388, 32.0903) -> (134.2871, 32.0903)
  line L139 (134.2871, 32.0903) -> (136.8668, 21.1542)
  spline S258 degree 2 poles (136.8668, 21.1542) (136.9439, 20.8676) (137.0321, 20.6471) knots 0 0 0 1 1 1
  spline S259 degree 2 poles (137.0321, 20.6471) (137.1203, 20.4707) (137.4069, 20.3605) knots 0 0 0 1 1 1
  spline S260 degree 2 poles (137.4069, 20.3605) (137.6495, 20.2502) (137.8369, 20.0518) (137.8369, 19.8754) knots 0 0 0 1 2 2 2
  spline S261 degree 2 poles (137.8369, 19.8754) (137.8369, 19.3903) (137.1093, 19.3903) knots 0 0 0 1 1 1
  line L140 (137.1093, 19.3903) -> (132.4681, 19.3903)
  spline S262 degree 2 poles (132.4681, 19.3903) (132.1924, 19.3903) (131.8507, 19.666) (131.8507, 19.8864) knots 0 0 0 1 2 2 2
  spline S263 degree 2 poles (131.8507, 19.8864) (131.8507, 20.0739) (132.005, 20.2613) (132.2586, 20.3936) knots 0 0 0 1 2 2 2
  spline S264 degree 2 poles (132.2586, 20.3936) (132.446, 20.4928) (132.6003, 20.7133) (132.6003, 20.8786) knots 0 0 0 1 2 2 2
  spline S265 degree 2 poles (132.6003, 20.8786) (132.6003, 21.044) (132.5673, 21.1653) knots 0 0 0 1 1 1
  line L141 (132.5673, 21.1653) -> (132.2696, 22.5102)
  line L142 (132.2696, 22.5102) -> (129.6789, 22.5102)
  line L143 (129.6789, 22.5102) -> (129.9325, 23.6127)
  line L144 (129.9325, 23.6127) -> (132.0161, 23.6127)
  line L145 (132.0161, 23.6127) -> (130.2963, 31.1753)
  line L146 (130.2963, 31.1753) -> (130.5388, 32.0903)
  line L147 (129.8884, 29.7201) -> (130.3624, 27.8019)
  line L148 (130.3624, 27.8019) -> (128.7198, 21.7936)
  spline S266 degree 2 poles (128.7198, 21.7936) (128.6426, 21.5291) (128.6426, 21.3086) knots 0 0 0 1 1 1
  spline S267 degree 2 poles (128.6426, 21.3086) (128.6426, 20.7243) (129.1938, 20.4707) knots 0 0 0 1 1 1
  line L149 (129.1938, 20.4707) -> (129.5135, 20.3164)
  spline S268 degree 2 poles (129.5135, 20.3164) (129.8222, 20.1841) (129.8222, 19.8534) knots 0 0 0 1 1 1
  spline S269 degree 2 poles (129.8222, 19.8534) (129.8222, 19.3903) (129.1497, 19.3903) knots 0 0 0 1 1 1
  line L150 (129.1497, 19.3903) -> (126.7905, 19.3903)
  spline S270 degree 2 poles (126.7905, 19.3903) (126.4378, 19.3903) (126.0409, 19.677) (126.0409, 19.9305) knots 0 0 0 1 2 2 2
  spline S271 degree 2 poles (126.0409, 19.9305) (126.0409, 20.1951) (126.4488, 20.3715) knots 0 0 0 1 1 1
  spline S272 degree 2 poles (126.4488, 20.3715) (126.8346, 20.5479) (127.1984, 20.8125) (127.3638, 21.044) knots 0 0 0 1 2 2 2
  spline S273 degree 2 poles (127.3638, 21.044) (127.6174, 21.4298) (127.7937, 22.0582) knots 0 0 0 1 1 1
  line L151 (127.7937, 22.0582) -> (129.8884, 29.7201)
  line L152 (143.6798, 19.3903) -> (139.5346, 19.3903)
  line L153 (139.5346, 19.3903) -> (139.2921, 19.3903)
  spline S274 degree 2 poles (139.2921, 19.3903) (138.9614, 19.3903) (138.5976, 19.6439) (138.5976, 19.8754) knots 0 0 0 1 2 2 2
  spline S275 degree 2 poles (138.5976, 19.8754) (138.5976, 20.2502) (138.9724, 20.3715) knots 0 0 0 1 1 1
  spline S276 degree 2 poles (138.9724, 20.3715) (139.2811, 20.4818) (139.3803, 20.5259) (139.4354, 20.614) knots 0 0 0 1 2 2 2
  spline S277 degree 2 poles (139.4354, 20.614) (139.5457, 20.7574) (139.5457, 21.0881) knots 0 0 0 1 1 1
  line L154 (139.5457, 21.0881) -> (139.5457, 30.3926)
  spline S278 degree 2 poles (139.5457, 30.3926) (139.5457, 30.7233) (139.4354, 30.8667) knots 0 0 0 1 1 1
  spline S279 degree 2 poles (139.4354, 30.8667) (139.3803, 30.9548) (139.2811, 30.9989) (138.9724, 31.0982) knots 0 0 0 1 2 2 2
  spline S280 degree 2 poles (138.9724, 31.0982) (138.5976, 31.2194) (138.5976, 31.6053) knots 0 0 0 1 1 1
  spline S281 degree 2 poles (138.5976, 31.6053) (138.5976, 31.8368) (138.9614, 32.0903) (139.2921, 32.0903) knots 0 0 0 1 2 2 2
  line L155 (139.2921, 32.0903) -> (139.5346, 32.0903)
  line L156 (139.5346, 32.0903) -> (143.6908, 32.0903)
  line L157 (143.6908, 32.0903) -> (144.0105, 32.0903)
  spline S282 degree 2 poles (144.0105, 32.0903) (144.4184, 32.0903) (144.5948, 31.9801) knots 0 0 0 1 1 1
  spline S283 degree 2 poles (144.5948, 31.9801) (144.8373, 31.8258) (144.8373, 31.5832) knots 0 0 0 1 1 1
  spline S284 degree 2 poles (144.8373, 31.5832) (144.8373, 31.1753) (144.3853, 31.0761) knots 0 0 0 1 1 1
  spline S285 degree 2 poles (144.3853, 31.0761) (144.0215, 30.9879) (143.8892, 30.9328) (143.8231, 30.8556) knots 0 0 0 1 2 2 2
  spline S286 degree 2 poles (143.8231, 30.8556) (143.6798, 30.6792) (143.6798, 30.3265) knots 0 0 0 1 1 1
  line L158 (143.6798, 30.3265) -> (143.6798, 19.3903)
  line L159 (144.4404, 19.3903) -> (144.4404, 20.4377)
  spline S287 degree 2 poles (144.4404, 20.4377) (144.8924, 20.5148) (145.4216, 20.7243) (145.6641, 20.9117) knots 0 0 0 1 2 2 2
  spline S288 degree 2 poles (145.6641, 20.9117) (146.061, 21.2204) (146.7115, 22.3008) (146.9099, 22.9622) knots 0 0 0 1 2 2 2
  spline S289 degree 2 poles (146.9099, 22.9622) (147.0642, 23.4693) (147.3068, 23.8001) (147.5493, 23.8001) knots 0 0 0 1 2 2 2
  spline S290 degree 2 poles (147.5493, 23.8001) (147.8139, 23.8001) (147.9352, 23.5906) knots 0 0 0 1 1 1
  spline S291 degree 2 poles (147.9352, 23.5906) (147.9903, 23.4804) (147.9903, 23.1717) knots 0 0 0 1 1 1
  line L160 (147.9903, 23.1717) -> (147.9903, 19.3903)
  line L161 (147.9903, 19.3903) -> (144.4404, 19.3903)
  line L162 (154.3072, 23.1055) -> (154.3072, 30.3926)
  spline S292 degree 2 poles (154.3072, 30.3926) (154.3072, 30.7233) (154.197, 30.8667) knots 0 0 0 1 1 1
  spline S293 degree 2 poles (154.197, 30.8667) (154.1418, 30.9548) (154.0426, 30.9989) (153.7339, 31.0982) knots 0 0 0 1 2 2 2
  spline S294 degree 2 poles (153.7339, 31.0982) (153.3591, 31.2194) (153.3591, 31.5943) knots 0 0 0 1 1 1
  spline S295 degree 2 poles (153.3591, 31.5943) (153.3591, 31.8368) (153.7229, 32.0903) (154.0536, 32.0903) knots 0 0 0 1 2 2 2
  line L163 (154.0536, 32.0903) -> (154.2962, 32.0903)
  line L164 (154.2962, 32.0903) -> (158.4523, 32.0903)
  line L165 (158.4523, 32.0903) -> (158.6949, 32.0903)
  line L166 (158.6949, 32.0903) -> (159.0256, 32.0573)
  spline S296 degree 2 poles (159.0256, 32.0573) (159.1799, 32.0022) (159.3894, 31.7596) (159.3894, 31.5943) knots 0 0 0 1 2 2 2
  spline S297 degree 2 poles (159.3894, 31.5943) (159.3894, 31.2194) (159.0146, 31.0982) knots 0 0 0 1 1 1
  spline S298 degree 2 poles (159.0146, 31.0982) (158.7059, 30.9989) (158.6067, 30.9548) (158.5516, 30.8667) knots 0 0 0 1 2 2 2
  spline S299 degree 2 poles (158.5516, 30.8667) (158.4413, 30.7233) (158.4413, 30.3926) knots 0 0 0 1 1 1
  line L167 (158.4413, 30.3926) -> (158.4413, 22.5874)
  spline S300 degree 2 poles (158.4413, 22.5874) (158.4413, 21.8047) (158.5295, 21.1763) (158.6508, 20.9227) knots 0 0 0 1 2 2 2
  spline S301 degree 2 poles (158.6508, 20.9227) (158.772, 20.6912) (159.0697, 20.4928) (159.4886, 20.3605) knots 0 0 0 1 2 2 2
  line L168 (159.4886, 20.3605) -> (159.4886, 19.1368)
  line L169 (159.4886, 19.1368) -> (159.2902, 19.1368)
  spline S302 degree 2 poles (159.2902, 19.1368) (158.0775, 19.1368) (157.2727, 19.3573) knots 0 0 0 1 1 1
  spline S303 degree 2 poles (157.2727, 19.3573) (156.3357, 19.5998) (154.9246, 20.592) (154.6269, 21.1983) knots 0 0 0 1 2 2 2
  spline S304 degree 2 poles (154.6269, 21.1983) (154.3072, 21.8598) (154.3072, 23.1055) knots 0 0 0 1 1 1
  line L170 (160.3485, 19.1368) -> (160.3485, 20.3605)
  spline S305 degree 2 poles (160.3485, 20.3605) (161.2746, 20.4818) (161.9029, 21.1212) knots 0 0 0 1 1 1
  spline S306 degree 2 poles (161.9029, 21.1212) (162.6085, 21.8598) (162.6085, 23.2268) knots 0 0 0 1 1 1
  line L171 (162.6085, 23.2268) -> (162.6085, 29.2902)
  spline S307 degree 2 poles (162.6085, 29.2902) (162.6085, 30.569) (161.6273, 31.0761) knots 0 0 0 1 1 1
  spline S308 degree 2 poles (161.6273, 31.0761) (161.3407, 31.2194) (161.1643, 31.4399) (161.1643, 31.6384) knots 0 0 0 1 2 2 2
  spline S309 degree 2 poles (161.1643, 31.6384) (161.1643, 31.8809) (161.5171, 32.0903) (161.925, 32.0903) knots 0 0 0 1 2 2 2
  line L172 (161.925, 32.0903) -> (164.196, 32.0903)
  spline S310 degree 2 poles (164.196, 32.0903) (164.4826, 32.0903) (164.6811, 32.0573) (164.7693, 32.0022) knots 0 0 0 1 2 2 2
  spline S311 degree 2 poles (164.7693, 32.0022) (165.0118, 31.8699) (165.0118, 31.6273) knots 0 0 0 1 1 1
  spline S312 degree 2 poles (165.0118, 31.6273) (165.0118, 31.4179) (164.8685, 31.2745) knots 0 0 0 1 1 1
  spline S313 degree 2 poles (164.8685, 31.2745) (164.8134, 31.2305) (164.4606, 31.032) knots 0 0 0 1 1 1
  spline S314 degree 2 poles (164.4606, 31.032) (164.0527, 30.8005) (163.5897, 29.8855) (163.5897, 29.2902) knots 0 0 0 1 2 2 2
  line L173 (163.5897, 29.2902) -> (163.5897, 23.2268)
  spline S315 degree 2 poles (163.5897, 23.2268) (163.5897, 21.6614) (162.9062, 20.6581) knots 0 0 0 1 1 1
  spline S316 degree 2 poles (162.9062, 20.6581) (162.399, 19.9085) (161.462, 19.4675) knots 0 0 0 1 1 1
  spline S317 degree 2 poles (161.462, 19.4675) (160.999, 19.236) (160.3485, 19.1368) knots 0 0 0 1 1 1
  line L174 (170.7003, 32.3439) -> (170.7003, 31.2745)
  spline S318 degree 2 poles (170.7003, 31.2745) (170.1271, 31.1092) (169.5207, 30.4477) (169.5207, 29.9737) knots 0 0 0 1 2 2 2
  spline S319 degree 2 poles (169.5207, 29.9737) (169.5207, 29.4996) (170.0279, 28.8051) (170.5901, 28.4854) knots 0 0 0 1 2 2 2
  spline S320 degree 2 poles (170.5901, 28.4854) (170.976, 28.2759) (172.354, 27.6696) knots 0 0 0 1 1 1
  spline S321 degree 2 poles (172.354, 27.6696) (173.1918, 27.3058) (174.1069, 26.7215) (174.5258, 26.2805) knots 0 0 0 1 2 2 2
  spline S322 degree 2 poles (174.5258, 26.2805) (175.6172, 25.134) (175.6172, 23.5355) knots 0 0 0 1 1 1
  spline S323 degree 2 poles (175.6172, 23.5355) (175.6172, 22.3449) (174.4266, 20.3495) (173.3903, 19.7762) knots 0 0 0 1 2 2 2
  spline S324 degree 2 poles (173.3903, 19.7762) (172.828, 19.4785) (171.4941, 19.1368) (170.9208, 19.1368) knots 0 0 0 1 2 2 2
  line L175 (170.9208, 19.1368) -> (170.9208, 20.1951)
  spline S325 degree 2 poles (170.9208, 20.1951) (171.7256, 20.3936) (172.4422, 21.0881) (172.4422, 21.6834) knots 0 0 0 1 2 2 2
  spline S326 degree 2 poles (172.4422, 21.6834) (172.4422, 22.3118) (171.8799, 22.7858) knots 0 0 0 1 1 1
  spline S327 degree 2 poles (171.8799, 22.7858) (171.5161, 23.0945) (170.4688, 23.5465) knots 0 0 0 1 1 1
  spline S328 degree 2 poles (170.4688, 23.5465) (169.3333, 24.0536) (168.4845, 24.4836) (168.0876, 24.7702) knots 0 0 0 1 2 2 2
  spline S329 degree 2 poles (168.0876, 24.7702) (166.3457, 26.016) (166.3457, 28.0885) knots 0 0 0 1 1 1
  spline S330 degree 2 poles (166.3457, 28.0885) (166.3457, 29.1469) (167.2167, 30.9438) (167.9994, 31.495) knots 0 0 0 1 2 2 2